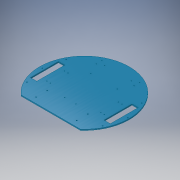
# Autodesk Inventor part: BottomPlate
Saved by Autodesk Inventor 2019 (Build 230136000, 136)
## iProperties
Created: 2019-09-28
Part Number: BottomPlate
Material: Generic
Document SubType Name: Modeling
Designer: james
Density: 1 g/cm^3
Appearance: Sky Blue Dark
Author: james
Autodesk Inventor part; units mm, degrees
ref_plane "YZ Plane" through (0, 0, 0) normal (1, 0, 0) x (0, 1, 0)
ref_plane "XZ Plane" through (0, 0, 0) normal (0, 1, 0) x (-1, 0, 0)
ref_plane "XY Plane" through (0, 0, 0) normal (0, 0, 1) x (1, 0, 0)
sketch "Sketch1" plane through (0, 0, 0) normal (0, 1, 0) x (-1, 0, 0)
  circle A0 centre (0, 0) radius 203.2
  dimension "d0" = 406.4
  constraints: 1 centre point, 1 coincident
  measures "d0" diameter of A0
extrude "Extrusion1" add sketch "Sketch1" along normal blind 4.7625
sketch "Sketch2" plane through (0, 4.7625, 0) normal (0, 1, 0) x (1, 0, 0)
  point P0 (0, 0)
  point P1 (114.3, 40.005)
  point P2 (114.3, -39.995)
  point P3 (-114.3, 40.005)
  point P4 (-114.3, -39.995)
  dimension "d3" = 0
  dimension "d4" = 80
  dimension "d5" = 40.005
  dimension "d6" = 0
  dimension "d7" = 0
  dimension "d8" = 0
  dimension "d9" = 114.3
  dimension "d10" = 114.3
  measures "d3" horizontal distance of point (-114.3, -39.995) point (-114.3, 40.005)
  measures "d4" distance of point (-114.3, -39.995) point (-114.3, 40.005)
  measures "d5" vertical distance of point (-114.3, 40.005) point (0, 0)
  measures "d6" vertical distance of point (-114.3, 40.005) point (114.3, 40.005)
  measures "d7" vertical distance of point (-114.3, -39.995) point (114.3, -39.995)
  measures "d8" horizontal distance of point (114.3, -39.995) point (114.3, 40.005)
  measures "d9" horizontal distance of point (0, 0) point (-114.3, 40.005)
  measures "d10" horizontal distance of point (114.3, 40.005) point (0, 0)
hole "Hole1" at (114.3, 4.7625, -40.005) at (114.3, 4.7625, 39.995) at (-114.3, 4.7625, -40.005) at (-114.3, 4.7625, 39.995) direction (0, -1, 0) diameter 3.175 end through all
sketch "Sketch3" plane through (0, 4.7625, 0) normal (0, 1, 0) x (1, 0, 0)
  line L0 (180.975, 63.5) -> (152.4, 63.5)
  line L1 (152.4, 63.5) -> (152.4, -63.5)
  line L2 (152.4, -63.5) -> (180.975, -63.5)
  line L3 (180.975, -63.5) -> (180.975, 63.5)
  line L4 (-152.4, 63.5) -> (-180.975, 63.5)
  line L5 (-180.975, 63.5) -> (-180.975, -63.5)
  line L6 (-180.975, -63.5) -> (-152.4, -63.5)
  line L7 (-152.4, -63.5) -> (-152.4, 63.5)
  point P0 (0, 0)
  dimension "d18" = 0
  dimension "d19" = 0
  dimension "d20" = 152.4
  dimension "d21" = 152.4
  dimension "d22" = 127
  dimension "d23" = 63.5
  dimension "d24" = 28.575
  dimension "d25" = 28.575
  constraints: 16 end point, 4 parallel, 2 horizontal, 2 perpendicular
  measures "d18" distance between parallel lines of L6 L2
  measures "d19" distance between parallel lines of L0 L4
  measures "d20" distance from line of point (0, 0) L7
  measures "d21" distance from line of L1 point (0, 0)
  measures "d22" distance of L2.end L0.start
  measures "d23" distance from line of point (0, 0) L0
  measures "d24" distance between parallel lines of L7 L5
  measures "d25" distance between parallel lines of L3 L1
extrude "Extrusion2" cut sketch "Sketch3" against normal blind 25.4
sketch "Sketch4" plane through (0, 4.7625, 0) normal (0, 1, 0) x (1, 0, 0)
  line L0 (152.4, -63.5) -> (152.4, 63.5) projected
  line L1 (152.4, 63.5) -> (180.975, 63.5) projected
  line L2 (180.975, 63.5) -> (180.975, -63.5) projected
  line L3 (180.975, -63.5) -> (152.4, -63.5) projected
  line L4 (-180.975, -63.5) -> (-180.975, 63.5) projected
  line L5 (-180.975, 63.5) -> (-152.4, 63.5) projected
  line L6 (-152.4, 63.5) -> (-152.4, -63.5) projected
  line L7 (-152.4, -63.5) -> (-180.975, -63.5) projected
  circle A0 centre (-114.3, 40.005) radius 1.5875 projected
  circle A1 centre (114.3, 40.005) radius 1.5875 projected
  circle A2 centre (114.3, -39.995) radius 1.5875 projected
  circle A3 centre (-114.3, -39.995) radius 1.5875 projected
  circle A4 centre (0, 0) radius 203.2 projected
  circle A5 centre (114.3, -39.995) radius 1.5875 projected
  point P0 (-130.302, 40.005)
  point P1 (-130.302, -39.995)
  point P2 (130.302, 40.005)
  point P3 (130.302, -39.995)
  dimension "d28" = 0
  dimension "d29" = 0
  dimension "d30" = 0
  dimension "d32" = 0
  dimension "d33" = 0
  dimension "d34" = 0
  dimension "d43" = 16.002
  dimension "d44" = 16.002
  measures "d28" horizontal distance of point (-130.302, 40.005) point (-130.302, -39.995)
  measures "d29" vertical distance of A0.centre point (-130.302, 40.005)
  measures "d30" vertical distance of A3.centre point (-130.302, -39.995)
  measures "d32" horizontal distance of point (130.302, 40.005) point (130.302, -39.995)
  measures "d33" vertical distance of A1.centre point (130.302, 40.005)
  measures "d34" vertical distance of point (130.302, -39.995) A2.centre
  measures "d43" distance of A5.centre point (130.302, -39.995)
  measures "d44" distance of point (-130.302, -39.995) A3.centre
hole "Hole2" at (-130.302, 4.7625, -40.005) at (-130.302, 4.7625, 39.995) at (130.302, 4.7625, -40.005) at (130.302, 4.7625, 39.995) direction (0, -1, 0) diameter 3.175 end through all
sketch "Sketch5" plane through (0, 4.7625, 0) normal (0, 1, 0) x (1, 0, 0)
  point P0 (0, 0)
  point P1 (60.325, 152.4)
  point P2 (60.325, 88.9)
  point P3 (-60.325, 88.9)
  point P4 (-60.325, 152.4)
  dimension "d45" = 0
  dimension "d46" = 0
  dimension "d47" = 0
  dimension "d48" = 0
  dimension "d49" = 60.325
  dimension "d50" = 60.325
  dimension "d51" = 63.5
  dimension "d52" = 88.9
  measures "d45" horizontal distance of point (60.325, 152.4) point (60.325, 88.9)
  measures "d46" horizontal distance of point (-60.325, 152.4) point (-60.325, 88.9)
  measures "d47" vertical distance of point (60.325, 88.9) point (-60.325, 88.9)
  measures "d48" vertical distance of point (-60.325, 152.4) point (60.325, 152.4)
  measures "d49" horizontal distance of point (0, 0) point (60.325, 88.9)
  measures "d50" horizontal distance of point (0, 0) point (-60.325, 152.4)
  measures "d51" distance of point (-60.325, 152.4) point (-60.325, 88.9)
  measures "d52" vertical distance of point (-60.325, 88.9) point (0, 0)
hole "Hole3" at (60.325, 4.7625, -152.4) at (60.325, 4.7625, -88.9) at (-60.325, 4.7625, -88.9) at (-60.325, 4.7625, -152.4) direction (0, -1, 0) diameter 3.175 end through all
sketch "Sketch6" plane through (0, 4.7625, 0) normal (0, 1, 0) x (1, 0, 0)
  circle A0 centre (60.325, 152.4) radius 1.5875 projected
  circle A1 centre (-60.325, 152.4) radius 1.5875 projected
  point P0 (0, 0)
  point P1 (-85.725, 139.7)
  point P2 (85.725, 139.7)
  point P3 (-85.725, 165.1)
  point P4 (85.725, 165.1)
  dimension "d64" = 0
  dimension "d65" = 25.4
  dimension "d66" = 0
  dimension "d67" = 25.4
  dimension "d68" = 12.7
  dimension "d69" = 25.4
  dimension "d70" = 12.7
  dimension "d71" = 25.4
  measures "d64" horizontal distance of point (-85.725, 139.7) point (-85.725, 165.1)
  measures "d65" distance of point (-85.725, 139.7) point (-85.725, 165.1)
  measures "d66" horizontal distance of point (85.725, 139.7) point (85.725, 165.1)
  measures "d67" distance of point (85.725, 139.7) point (85.725, 165.1)
  measures "d68" vertical distance of point (-85.725, 139.7) A1.centre
  measures "d69" horizontal distance of A1.centre point (-85.725, 139.7)
  measures "d70" vertical distance of A0.centre point (85.725, 139.7)
  measures "d71" horizontal distance of A0.centre point (85.725, 139.7)
hole "Hole4" at (-85.725, 4.7625, -139.7) at (85.725, 4.7625, -139.7) at (-85.725, 4.7625, -165.1) at (85.725, 4.7625, -165.1) direction (0, -1, 0) diameter 3.175 end through all
sketch "Sketch8" plane through (0, 4.7625, 0) normal (0, 1, 0) x (1, 0, 0)
  line L0 (-76.2, 0) -> (-76.2, -101.6) projected
  line L1 (-76.2, -101.6) -> (76.2, -101.6) projected
  point P0 (0, 0)
  point P1 (-25.4, -63.5)
  point P2 (25.4, -63.5)
  point P3 (-203.2, 0)
  dimension "d86" = 0
  dimension "d89" = 50.8
  dimension "d99" = 63.5
  dimension "d100" = 25.4
  measures "d86" vertical distance of point (25.4, -63.5) point (-25.4, -63.5)
  measures "d89" distance of point (-25.4, -63.5) point (25.4, -63.5)
  measures "d99" vertical distance of point (25.4, -63.5) point (0, 0)
  measures "d100" horizontal distance of point (25.4, -63.5) point (0, 0)
hole "Hole5" at (-25.4, 4.7625, 63.5) at (25.4, 4.7625, 63.5) direction (0, -1, 0) diameter 3.175 depth 25.4 tip angle 118.188
sketch "Sketch9" plane through (0, 4.7625, 0) normal (0, 1, 0) x (1, 0, 0)
  line L0 (-76.2, -158.75) -> (76.2, -158.75)
  line L1 (76.2, -158.75) -> (76.2, -299.4145)
  line L2 (76.2, -299.4145) -> (-76.2, -299.4145)
  line L3 (-76.2, -299.4145) -> (-76.2, -158.75)
  point P0 (0, 0)
  dimension "d101" = 158.75
  dimension "d104" = 76.2
  dimension "d105" = 76.2
  constraints: 8 end point, 2 parallel, 1 horizontal, 1 perpendicular
  measures "d101" distance from line of point (0, 0) L0
  measures "d104" distance from line of L1 point (0, 0)
  measures "d105" distance from line of point (0, 0) L3
extrude "Extrusion4" cut sketch "Sketch9" against normal blind 25.4
sketch "Sketch10" plane through (0, 4.7625, 0) normal (0, 1, 0) x (1, 0, 0)
  circle A0 centre (25.4, -63.5) radius 1.5875 projected
  point P0 (0, 0)
  point P1 (-92.075, -76.2)
  point P2 (-92.075, -127)
  point P3 (92.075, -76.2)
  point P4 (92.075, -127)
  dimension "d106" = 0
  dimension "d107" = 0
  dimension "d108" = 0
  dimension "d109" = 50.8
  dimension "d110" = 0
  dimension "d111" = 92.075
  dimension "d112" = 92.075
  dimension "d113" = 12.7
  measures "d106" horizontal distance of point (92.075, -127) point (92.075, -76.2)
  measures "d107" vertical distance of point (-92.075, -76.2) point (92.075, -76.2)
  measures "d108" horizontal distance of point (-92.075, -127) point (-92.075, -76.2)
  measures "d109" distance of point (-92.075, -127) point (-92.075, -76.2)
  measures "d110" vertical distance of point (92.075, -127) point (-92.075, -127)
  measures "d111" horizontal distance of point (0, 0) point (92.075, -76.2)
  measures "d112" horizontal distance of point (-92.075, -76.2) point (0, 0)
  measures "d113" vertical distance of point (92.075, -76.2) A0.centre
hole "Hole6" at (-92.075, 4.7625, 76.2) at (-92.075, 4.7625, 127) at (92.075, 4.7625, 76.2) at (92.075, 4.7625, 127) direction (0, -1, 0) diameter 4.4958 end through all clearance for "Flat Head Machine Screw (82)" size "#8" standard "Ansi Unified Screw Threads"
sketch "Sketch11" plane through (0, 4.7625, 0) normal (0, 1, 0) x (1, 0, 0)
  line L0 (-208.3866, -152.4) -> (200.3636, -152.4)
  line L1 (200.3636, -152.4) -> (200.3636, -247.6891)
  line L2 (200.3636, -247.6891) -> (-208.3866, -247.6891)
  line L3 (-208.3866, -247.6891) -> (-208.3866, -152.4)
  circle A0 centre (-92.075, -127) radius 2.2479 projected
  point P0 (0, 0)
  dimension "d121" = 25.4
  constraints: 8 end point, 2 parallel, 1 horizontal, 1 perpendicular
  measures "d121" distance from line of L0 A0.centre
extrude "Extrusion5" cut sketch "Sketch11" against normal blind 25.4 contours L0 L1 L2 L3
sketch "Sketch12" plane through (0, 4.7625, 0) normal (0, 1, 0) x (1, 0, 0)
  point P0 (0, 0)
  point P1 (196.85, 0)
  point P2 (171.45, 88.9)
  point P3 (171.45, -88.9)
  point P4 (-171.45, -88.9)
  point P5 (-190.5, 0)
  point P6 (-171.45, 88.9)
  dimension "d124" = 0
  dimension "d125" = 88.9
  dimension "d126" = 88.9
  dimension "d127" = 171.45
  dimension "d128" = 171.45
  dimension "d129" = 171.45
  dimension "d130" = 171.45
  dimension "d131" = 88.9
  dimension "d132" = 88.9
  dimension "d133" = 0
  dimension "d134" = 196.85
  dimension "d142" = 190.5
  measures "d124" vertical distance of point (-190.5, 0) point (0, 0)
  measures "d125" vertical distance of point (-171.45, 88.9) point (0, 0)
  measures "d126" vertical distance of point (-171.45, -88.9) point (0, 0)
  measures "d127" horizontal distance of point (-171.45, -88.9) point (0, 0)
  measures "d128" horizontal distance of point (0, 0) point (-171.45, 88.9)
  measures "d129" horizontal distance of point (171.45, 88.9) point (0, 0)
  measures "d130" horizontal distance of point (0, 0) point (171.45, -88.9)
  measures "d131" vertical distance of point (0, 0) point (171.45, -88.9)
  measures "d132" vertical distance of point (0, 0) point (171.45, 88.9)
  measures "d133" vertical distance of point (0, 0) point (196.85, 0)
  measures "d134" distance of point (0, 0) point (196.85, 0)
  measures "d142" distance of point (0, 0) point (-190.5, 0)
hole "Hole7" at (196.85, 4.7625, 0) at (171.45, 4.7625, -88.9) at (171.45, 4.7625, 88.9) at (-171.45, 4.7625, 88.9) at (-190.5, 4.7625, 0) at (-171.45, 4.7625, -88.9) direction (0, -1, 0) diameter 4.4958 end through all clearance for "Flat Head Machine Screw (82)" size "#8" standard "Ansi Unified Screw Threads"
body "Solid1"
